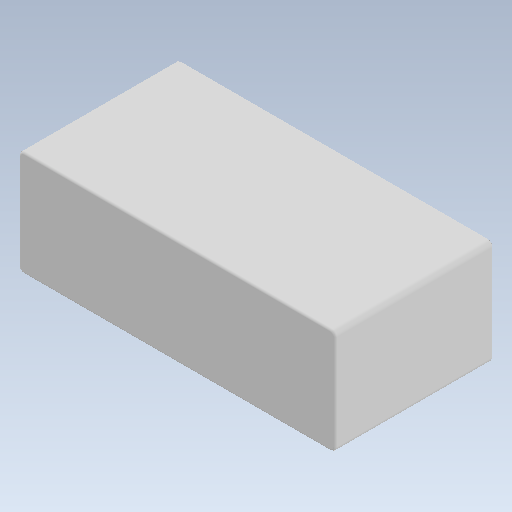
# Autodesk Inventor part: body
Saved by Autodesk Inventor 2020 (Build 240168000, 168)
## iProperties
Created: 2022-12-14
Part Number: body
Material: Generic
Document SubType Name: Modeling
Designer: Manish
Density: 1 g/cm^3
Appearance: Default
Author: Manish
Autodesk Inventor part; units mm, degrees
ref_plane "YZ Plane" through (0, 0, 0) normal (1, 0, 0) x (0, 1, 0)
ref_plane "XZ Plane" through (0, 0, 0) normal (0, 1, 0) x (-1, 0, 0)
ref_plane "XY Plane" through (0, 0, 0) normal (0, 0, 1) x (1, 0, 0)
sketch "Sketch1" plane through (0, 0, 0) normal (0, 0, 1) x (1, 0, 0)
  line L0 (0, 5) -> (0, 95)
  line L1 (5, 100) -> (295, 100)
  line L2 (300, 95) -> (300, 5)
  line L3 (295, 0) -> (5, 0)
  arc A0 (5, 100) -> (0, 95) centre (5, 95) ccw
  arc A1 (0, 5) -> (5, 0) centre (5, 5) ccw
  arc A2 (295, 0) -> (300, 5) centre (295, 5) ccw
  arc A3 (300, 95) -> (295, 100) centre (295, 95) ccw
  line L4 (295, 95) -> (5, 95)
  line L5 (5, 95) -> (5, 5)
  line L6 (5, 5) -> (295, 5)
  line L7 (295, 5) -> (295, 95)
  point P0 (0, 0)
  point P1 (0, 100)
  point P2 (300, 100)
  dimension "d0" = 100
  dimension "d1" = 300
  dimension "d2" = 5
  dimension "d6" = 5
  constraints: 16 end point, 8 point on circle, 8 tangent, 6 point on line, 4 centre point, 4 parallel, 3 equal radius, 2 perpendicular, 1 vertical, 3 other
  measures "d0" distance of point (0, 0) point (0, 100)
  measures "d1" distance of point (0, 100) point (300, 100)
  measures "d2" radius of A0
  measures "d6" distance between parallel lines of L1 L4
extrude "Extrusion1" add sketch "Sketch1" along normal blind 150 contours L0 A0 L1 A3 L2 A2 L3 A1 | L7 L6 L5 L4
fillet "Fillet1" radius 2 16 edges at (298.5355, 98.5355, 150) (150, 100, 150) (1.4645, 98.5355, 150) (0, 50, 150) (1.4645, 1.4645, 150) (150, 0, 150) (298.5355, 1.4645, 150) (300, 50, 150) (298.5355, 98.5355, 0) (150, 100, 0) (1.4645, 98.5355, 0) (0, 50, 0) (1.4645, 1.4645, 0) (150, 0, 0) (298.5355, 1.4645, 0) (300, 50, 0)
body "Solid1"
